模型架子 (Autodesk Fusion 360 design; units mm, degrees)
part number: 2026-05-04-18-34-39-242
Autodesk Fusion 360 part; units mm, degrees
sketch "草图2" plane through (0, 0, 0) normal (0, 0, 1) x (1, 0, 0)
  line L0 (68, 55) -> (-68, 55)
  line L1 (-70, 53) -> (-70, -53)
  line L2 (-68, -55) -> (68, -55)
  line L3 (70, -53) -> (70, 53)
  line L4 (70, 55) -> (-70, -55) construction
  line L5 (-70, 55) -> (70, -55) construction
  arc A0 (70, 53) -> (68, 55) centre (68, 53) ccw
  arc A1 (68, -55) -> (70, -53) centre (68, -53) ccw
  arc A2 (-70, -53) -> (-68, -55) centre (-68, -53) ccw
  arc A3 (-68, 55) -> (-70, 53) centre (-68, 53) ccw
  line L6 (-68, -58) -> (68, -58)
  line L7 (73, -53) -> (73, 53)
  line L8 (68, 58) -> (-68, 58)
  line L9 (-73, 53) -> (-73, -53)
  line L10 (-73, 58) -> (73, 58)
  line L11 (73, 58) -> (73, -58)
  line L12 (73, -58) -> (-73, -58)
  line L13 (-73, -58) -> (-73, 58)
  dimension "d11" = 140
  dimension "d12" = 110
  dimension "d14" = 2
  dimension "d15" = 116
  dimension "d16" = 146
  constraint horizontal L0
  constraint perpendicular L0 L1
  constraint parallel L0 L2
  constraint parallel L1 L3
  constraint coincident L4 origin
  constraint coincident L5 origin
  constraint coincident L4.start L0
  constraint coincident L4.start L3
  constraint tangent L0 A0
  constraint tangent L3 A0
  constraint coincident L5.end L3
  constraint coincident L5.end L2
  constraint tangent L3 A1
  constraint tangent L2 A1
  constraint equal A0 A1
  constraint coincident L4.end L1
  constraint coincident L4.end L2
  constraint tangent L1 A2
  constraint tangent L2 A2
  constraint equal A0 A2
  constraint coincident L5.start L0
  constraint coincident L5.start L1
  constraint tangent L0 A3
  constraint tangent L1 A3
  constraint equal A0 A3
  constraint horizontal L10
  constraint vertical L11
  constraint horizontal L12
  constraint vertical L13
  measures "d11" distance of L4.end L5.end
  measures "d12" distance of L5.start L4.end
  measures "d14" radius of A0
  measures "d15" distance of L6 L8
  measures "d16" distance of L7 L9
extrude "拉伸1" add sketch "草图2" along normal blind 100
fillet "圆角1" radius 3 8 edges at (70, 0, 100) (69.4142, -54.4142, 100) (0, -55, 100) (-69.4142, -54.4142, 100) (-70, 0, 100) (-69.4142, 54.4142, 100) (0, 55, 100) (69.4142, 54.4142, 100)
